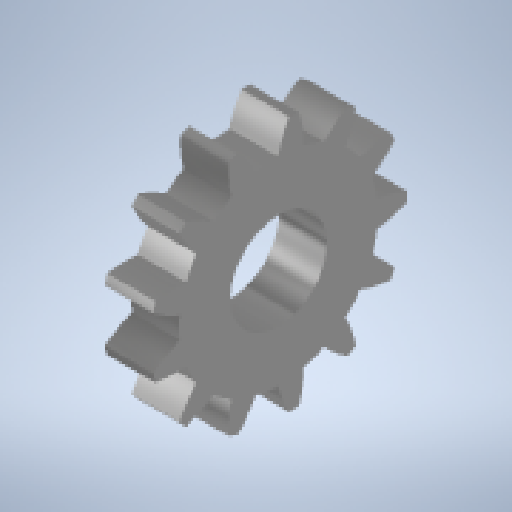
# Autodesk Inventor part: Zahnrad_für_Kettenzug
Saved by Autodesk Inventor 2025.2 (Build 292293000, 293)
## iProperties
Created: 2025-02-03
Part Number: Zahnrad_für_Kettenzug
Material: Generisch
Document SubType Name: Modeling
Designer: unter
Density: 1 g/cm^3
Appearance: Vorgabe
Author: unter
Autodesk Inventor part; units mm, degrees
ref_plane "YZ Plane" through (0, 0, 0) normal (1, 0, 0) x (0, 1, 0)
ref_plane "XZ Plane" through (0, 0, 0) normal (0, 1, 0) x (-1, 0, 0)
ref_plane "XY Plane" through (0, 0, 0) normal (0, 0, 1) x (1, 0, 0)
derived "Skelett_Laufkatze.ipt"
sketch "Zahnrad_Zahnrad_seite" plane through (-131, 0, 62.4) normal (0, 0, -1) x (-1, 0, 0)
  line L0 (0, 0) -> (-2, 0) construction
  line L1 (-2, 0) -> (-17, 0)
  line L2 (-2, 15) -> (-17, 15)
  line L3 (-17, 15) -> (-17, 40)
  line L4 (-17, 40) -> (-2, 40)
  line L5 (-2, 40) -> (-2, 15)
  point P0 (-131, 0)
sketch "Zahnrad_Zahnrad_front" plane through (-129, 0, 62.4) normal (1, 0, 0) x (0, 1, 0)
  circle A0 centre (0, 0) radius 15
  circle A1 centre (0, 0) radius 40
  circle A2 centre (0, 0) radius 31 construction
  line L0 (0, 0) -> (0, 40) construction
  arc A3 (8.1226, 39.1666) -> (3.4104, 30.8118) centre (34.9342, 18.5381) ccw
  arc A4 (-3.4104, 30.8118) -> (-8.1226, 39.1666) centre (-34.9342, 18.5381) ccw
  arc A5 (3.4104, 30.8118) -> (-3.4104, 30.8118) centre (0, 0) ccw
  circle A6 centre (0, 0) radius 36
  point P0 (0, -62.4)
  point P1 (15, 0)
  point P2 (40, 0)
revolve "Rohling_Zahnrad" add sketch "Zahnrad_Zahnrad_seite" angle 360 about axis through (-129, 0, 62.4) along (1, 0, 0)
extrude "Zahngeometrie" cut sketch "Zahnrad_Zahnrad_front" along normal through all contours A3 A6 A4 A1 | A3 A5 A4 A6 picked at (0.6348, 38.5879) picked at (-0.3796, 34.2927)
pattern_circular "Anzahl_zähne" count 13 over 360 about axis through (-121.5, 0, 62.4) along (1, 0, 0) of "Zahngeometrie"
